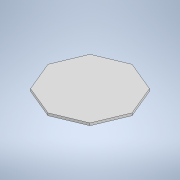
# Autodesk Inventor part: Support haut
Saved by Autodesk Inventor 2020 (Build 240168000, 168)
## iProperties
Created: 2019-11-28
Part Number: Support haut
Material: Générique
Document SubType Name: Modeling
Designer: erwan
Density: 1 g/cm^3
Appearance: Par défaut
Author: erwan
Autodesk Inventor part; units mm, degrees
ref_plane "YZ Plane" through (0, 0, 0) normal (1, 0, 0) x (0, 1, 0)
ref_plane "XZ Plane" through (0, 0, 0) normal (0, 1, 0) x (-1, 0, 0)
ref_plane "XY Plane" through (0, 0, 0) normal (0, 0, 1) x (1, 0, 0)
sketch "Esquisse1" plane through (0, 0, 0) normal (0, 1, 0) x (-1, 0, 0)
  line L0 (0, -175) -> (123.7437, -123.7437)
  line L1 (123.7437, -123.7437) -> (175, 0)
  line L2 (175, 0) -> (123.7437, 123.7437)
  line L3 (123.7437, 123.7437) -> (0, 175)
  line L4 (0, 175) -> (-123.7437, 123.7437)
  line L5 (-123.7437, 123.7437) -> (-175, 0)
  line L6 (-175, 0) -> (-123.7437, -123.7437)
  line L7 (-123.7437, -123.7437) -> (0, -175)
  point P0 (0, 0)
  constraints: 16 end point, 3 perpendicular
extrude "Extrusion1" add sketch "Esquisse1" along normal blind 10
